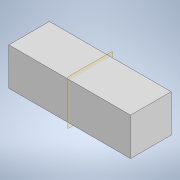
# Autodesk Inventor part: Block
Saved by Autodesk Inventor 2020 (Build 240168000, 168)
## iProperties
Created: 2019-12-31
Part Number: Block
Material: Générique
Document SubType Name: Modeling
Designer: damien
Density: 1 g/cm^3
Appearance: Par défaut
Author: damien
Autodesk Inventor part; units mm, degrees
ref_plane "YZ Plane" through (0, 0, 0) normal (1, 0, 0) x (0, 1, 0)
ref_plane "XZ Plane" through (0, 0, 0) normal (0, 1, 0) x (-1, 0, 0)
ref_plane "XY Plane" through (0, 0, 0) normal (0, 0, 1) x (1, 0, 0)
sketch "Esquisse1" plane through (0, 0, 0) normal (1, 0, 0) x (0, 1, 0)
  line L0 (-9.275, -10) -> (9.275, -10)
  line L1 (9.275, -10) -> (9.275, 10)
  line L2 (9.275, 10) -> (-9.275, 10)
  line L3 (-9.275, 10) -> (-9.275, -10)
  line L4 (-9.275, -10) -> (9.275, 10) construction
  line L5 (9.275, -10) -> (-9.275, 10) construction
  point P0 (0, 0)
  dimension "d0" = 20
  dimension "d1" = 18.55
  constraints: 12 end point, 2 midpoint, 2 parallel, 1 horizontal, 1 perpendicular
  measures "d0" distance of L2.end L0.start
  measures "d1" distance of L0.start L0.end
extrude "Extrusion1" add sketch "Esquisse1" along normal blind 60
ref_plane "Plan de construction1" through (30, 0, 0) normal (1, 0, 0) x (0, 0, -1)
